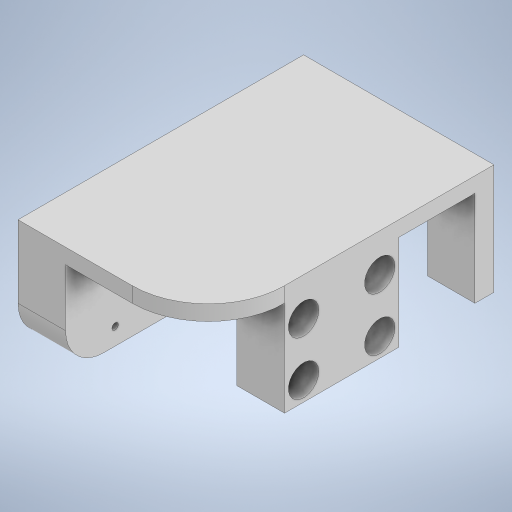
# Autodesk Inventor part: モーター接続
Saved by Autodesk Inventor 2024.1 (Build 281209000, 209)
## iProperties
Created: 2024-04-01
Part Number: モーター接続
Material: 一般
Document SubType Name: Modeling
Designer: hibik
Density: 1 g/cm^3
Appearance: 既定
Author: hibik
Autodesk Inventor part; units mm, degrees
ref_plane "YZ Plane" through (0, 0, 0) normal (1, 0, 0) x (0, 1, 0)
ref_plane "XZ Plane" through (0, 0, 0) normal (0, 1, 0) x (-1, 0, 0)
ref_plane "XY Plane" through (0, 0, 0) normal (0, 0, 1) x (1, 0, 0)
sketch "スケッチ1" plane through (0, 0, 0) normal (0, 1, 0) x (-1, 0, 0)
  line L0 (0, 0) -> (50, 0)
  line L1 (50, 0) -> (50, -75)
  line L2 (50, -75) -> (0, -75)
  line L3 (0, -75) -> (0, 0)
  dimension "d0" = 50
  dimension "d1" = 75
  constraints: 8 end point, 2 parallel, 1 horizontal, 1 perpendicular
  measures "d0" distance of L1.end L2.end
  measures "d1" distance of L0.end L1.end
extrude "押し出し1" add sketch "スケッチ1" along normal blind 29
sketch "スケッチ2" plane through (0, 0, 0) normal (0, -1, 0) x (1, 0, 0)
  line L0 (-50, 0) -> (0, 0) projected
  line L1 (0, -75) -> (-50, -75) projected
  line L2 (-37.5, 0) -> (-12.5, 0)
  line L3 (-12.5, 0) -> (-12.5, -75)
  line L4 (-12.5, -75) -> (-37.5, -75)
  line L5 (-37.5, -75) -> (-37.5, 0)
  line L6 (-50, 0) -> (0, 0) projected
  point P0 (-12.5, -37.5)
  point P1 (-25, 0)
  point P2 (-25, 0)
  dimension "d4" = 25
  constraints: 8 end point, 5 midpoint, 2 parallel, 2 point on line, 1 horizontal, 1 perpendicular
  measures "d4" distance from line of point (-12.5, -37.5) L5
extrude "押し出し2" cut sketch "スケッチ2" against normal blind 25
sketch "スケッチ3" plane through (0, 0, 0) normal (1, 0, 0) x (0, 0, -1)
  line L0 (0, 0) -> (20, 0)
  line L1 (20, 0) -> (20, 25)
  line L2 (20, 25) -> (0, 25)
  line L3 (0, 25) -> (0, 0)
  line L4 (50, 0) -> (70, 0)
  line L5 (70, 0) -> (70, 25)
  line L6 (70, 25) -> (50, 25)
  line L7 (50, 25) -> (50, 0)
  line L8 (0, 25) -> (75, 25) projected
  point P0 (60, 25)
  point P1 (10, 25)
  dimension "d7" = 20
  dimension "d8" = 20
  dimension "d9" = 50
  constraints: 16 end point, 4 parallel, 2 collinear, 2 horizontal, 2 midpoint, 2 perpendicular, 1 point on line
  measures "d7" distance between parallel lines of L1 L3
  measures "d8" distance between parallel lines of L5 L7
  measures "d9" distance of point (60, 25) point (10, 25)
extrude "押し出し3" cut sketch "スケッチ3" against normal up to surface (12.5 mm away)
sketch "スケッチ4" plane through (-50, 0, -75) normal (-1, 0, 0) x (0, 0, 1)
  circle A0 centre (62, 20.5) radius 0.85
  circle A1 centre (62, 4.5) radius 0.85
  circle A2 centre (11, 4.5) radius 0.85
  line L0 (62, 20.5) -> (62, 4.5) construction
  line L1 (62, 4.5) -> (11, 4.5) construction
  line L2 (75, 0) -> (75, 25) projected
  point P0 (75, 12.5)
  point P1 (62, 12.5)
  dimension "d12" = 1.7
  dimension "d13" = 1.7
  dimension "d14" = 1.7
  dimension "d15" = 16
  dimension "d16" = 51
  dimension "d17" = 13
  constraints: 4 end point, 3 centre point, 2 midpoint, 1 horizontal alignment, 1 perpendicular, 1 vertical
  measures "d12" diameter of A0
  measures "d13" diameter of A1
  measures "d14" diameter of A2
  measures "d15" distance of L0.start L0.end
  measures "d16" distance of L0.end L1.end
  measures "d17" distance between parallel lines of L2 L0
extrude "押し出し4" cut sketch "スケッチ4" against normal up to surface (12.5 mm away)
sketch "スケッチ5" plane through (-50, 0, -75) normal (-1, 0, 0) x (0, 0, 1)
  circle A0 centre (11, 4.5) radius 0.85 projected
  circle A1 centre (11, 4.5) radius 4
  circle A2 centre (62, 20.5) radius 0.85 projected
  circle A3 centre (62, 20.5) radius 4
  circle A4 centre (62, 4.5) radius 0.85 projected
  circle A5 centre (62, 4.5) radius 4
  point P0 (75, 0)
  dimension "d20" = 8
  dimension "d21" = 8
  dimension "d22" = 8
  constraints: 3 centre point, 3 coincident
  measures "d20" diameter of A1
  measures "d21" diameter of A3
  measures "d22" diameter of A5
extrude "押し出し5" cut sketch "スケッチ5" against normal blind 9
fillet "フィレット1" radius 10 2 edges at (-43.75, 0, 0) (-43.75, 0, -75)
sketch "スケッチ7" plane through (0, 0, -75) normal (1, 0, 0) x (0, 0, -1)
  line L0 (-30, 5) -> (-50, 5) construction
  line L1 (-50, 5) -> (-50, 19) construction
  line L2 (-50, 19) -> (-30, 19) construction
  line L3 (-30, 19) -> (-30, 5) construction
  line L4 (-55, 0) -> (-25, 0) projected
  line L5 (-25, 0) -> (-25, 25) projected
  line L6 (-55, 25) -> (-55, 0) projected
  line L7 (-75, 29) -> (0, 29) projected
  circle A0 centre (-50, 5) radius 1.35
  circle A1 centre (-30, 5) radius 1.35
  circle A2 centre (-30, 19) radius 1.35
  circle A3 centre (-50, 19) radius 1.35
  point P0 (-75, 0)
  dimension "d26" = 5
  dimension "d27" = 5
  dimension "d28" = 5
  dimension "d29" = 10
  dimension "d30" = 2.7
  dimension "d31" = 2.7
  dimension "d32" = 2.7
  dimension "d33" = 2.7
  constraints: 8 end point, 4 centre point, 4 coincident, 2 parallel, 1 horizontal, 1 perpendicular
  measures "d26" distance between parallel lines of L4 L0
  measures "d27" distance between parallel lines of L5 L3
  measures "d28" distance between parallel lines of L6 L1
  measures "d29" distance between parallel lines of L7 L2
  measures "d30" diameter of A0
  measures "d31" diameter of A1
  measures "d32" diameter of A2
  measures "d33" diameter of A3
extrude "押し出し6" cut sketch "スケッチ7" against normal through all
fillet "フィレット2" radius 20 1 edges at (0, 27, 0)
sketch "スケッチ8" plane through (0, 0, -75) normal (1, 0, 0) x (0, 0, -1)
  circle A0 centre (-30, 19) radius 4
  circle A1 centre (-30, 5) radius 4
  circle A2 centre (-50, 5) radius 4
  circle A3 centre (-50, 19) radius 4
  circle A4 centre (-30, 5) radius 1.35 projected
  circle A5 centre (-30, 19) radius 1.35 projected
  circle A6 centre (-50, 19) radius 1.35 projected
  circle A7 centre (-50, 5) radius 1.35 projected
  point P0 (-75, 0)
  dimension "d37" = 8
  dimension "d38" = 8
  dimension "d39" = 8
  dimension "d40" = 8
  constraints: 4 centre point, 4 concentric
  measures "d37" diameter of A0
  measures "d38" diameter of A1
  measures "d39" diameter of A2
  measures "d40" diameter of A3
extrude "押し出し7" cut sketch "スケッチ8" against normal blind 8 contours A0 | A1 | A2 | A3 | A4 | A5 | A6 | A7
sketch "スケッチ9" plane through (-50, 29, -75) normal (-1, 0, 0) x (0, 0, 1)
  circle A0 centre (30, -24) radius 4
  circle A1 centre (30, -10) radius 4
  circle A2 centre (50, -24) radius 4
  circle A3 centre (50, -10) radius 4
  circle A4 centre (30, -10) radius 1.35 projected
  circle A5 centre (30, -24) radius 1.35 projected
  circle A6 centre (50, -10) radius 1.35 projected
  circle A7 centre (50, -24) radius 1.35 projected
  point P0 (75, -29)
  dimension "d43" = 8
  dimension "d44" = 8
  dimension "d45" = 8
  dimension "d46" = 8
  constraints: 4 centre point, 4 concentric
  measures "d43" diameter of A0
  measures "d44" diameter of A1
  measures "d45" diameter of A2
  measures "d46" diameter of A3
extrude "押し出し8" cut sketch "スケッチ9" against normal blind 8 contours A0 | A1 | A2 | A3 | A4 | A5 | A6 | A7
equation "\"d8\" = d7"
